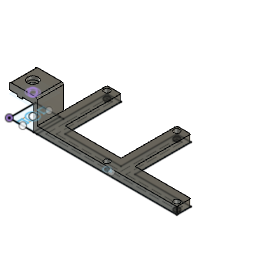
Micron_4010_Bed_FAN v2 (Autodesk Fusion 360 design; units mm, degrees)
Autodesk Fusion 360 part; units mm, degrees
sketch "Skizze1" plane through (0, 0, 0) normal (0, 0, 1) x (1, 0, 0)
  line L0 (0, 0) -> (0, 15)
  line L1 (0, 15) -> (14, 15)
  line L2 (14, 15) -> (14, 0)
  line L3 (14, 0) -> (0, 0)
  line L4 (14, 15) -> (16, 15)
  line L5 (14, 0) -> (16, 0)
  line L6 (16, 15) -> (16, 0)
  line L7 (16, 0) -> (96, 0)
  line L8 (96, 0) -> (96, 8)
  line L9 (16, 15) -> (16, 40)
  line L10 (16, 40) -> (24, 40)
  line L11 (24, 40) -> (24, 8)
  line L12 (24, 8) -> (56, 8)
  line L13 (56, 8) -> (56, 40)
  line L14 (56, 40) -> (64, 40)
  line L15 (64, 40) -> (64, 8)
  line L16 (64, 8) -> (96, 8)
  line L17 (18.5, 15) -> (18.5, 2.5) construction
  line L18 (18.5, 2.5) -> (93.5, 2.5) construction
  line L19 (93.5, 2.5) -> (93.5, 5.5) construction
  line L20 (61.5, 5.5) -> (93.5, 5.5) construction
  line L21 (61.5, 37.5) -> (61.5, 5.5) construction
  line L22 (58.5, 37.5) -> (61.5, 37.5) construction
  line L23 (58.5, 5.5) -> (58.5, 37.5) construction
  line L24 (21.5, 5.5) -> (58.5, 5.5) construction
  line L25 (21.5, 37.5) -> (21.5, 5.5) construction
  line L26 (18.5, 37.5) -> (21.5, 37.5) construction
  line L27 (18.5, 15) -> (18.5, 37.5) construction
  circle A0 centre (18.5, 37.5) radius 1.675
  circle A1 centre (58.5, 37.5) radius 1.675
  circle A2 centre (93.5, 2.5) radius 1.675
  line L28 (4.25, 0) -> (4.25, 15) construction
  line L29 (7.75, 0) -> (7.75, 15) construction
  line L30 (4.25, 0) -> (7.75, 0)
  line L31 (7.75, 0) -> (7.75, 3)
  line L32 (7.75, 3) -> (4.25, 3)
  line L33 (4.25, 3) -> (4.25, 0)
  line L34 (4.25, 15) -> (7.75, 15)
  line L35 (7.75, 15) -> (7.75, 12)
  line L36 (7.75, 12) -> (4.25, 12)
  line L37 (4.25, 12) -> (4.25, 15)
  circle A3 centre (6, 7.5) radius 1.5
  circle A4 centre (6, 7.5) radius 3
  line L38 (56, 2.5) -> (53.5, 2.5)
  circle A5 centre (53.5, 2.5) radius 1.675
  dimension "d1" = 15
  dimension "d2" = 14
  dimension "d3" = 2
  dimension "d4" = 2
  dimension "d5" = 80
  dimension "d6" = 8
  dimension "d7" = 90
  dimension "d8" = 25
  dimension "d9" = 90
  dimension "d10" = 8
  dimension "d11" = 32
  dimension "d12" = 32
  dimension "d13" = 32
  dimension "d14" = 8
  dimension "d15" = 90
  dimension "d16" = 32
  dimension "d17" = -2.5
  dimension "d18" = 3.35
  dimension "d20" = 3.35
  dimension "d21" = 3.35
  dimension "d26" = 3.5
  dimension "d27" = 3
  dimension "d28" = 3.5
  dimension "d29" = 3
  dimension "d30" = 3
  dimension "d31" = 6
  dimension "d64" = 2.5
  dimension "d65" = 3.35
  constraint coincident L0.start L3.end
  constraint vertical L0
  constraint perpendicular L0 L1
  constraint perpendicular L1 L2
  constraint perpendicular L0 L3
  constraint perpendicular L2 L4
  constraint perpendicular L2 L5
  constraint perpendicular L6 L7
  constraint perpendicular L4 L9
  constraint perpendicular L10 L11
  constraint perpendicular L11 L12
  constraint perpendicular L12 L13
  constraint perpendicular L14 L15
  constraint coincident L26.start L27.end
  constraint coincident L22.start L23.end
  constraint coincident L18.end L19.start
  constraint horizontal L30
  constraint vertical L31
  constraint horizontal L32
  constraint vertical L33
  constraint horizontal L34
  constraint vertical L35
  constraint horizontal L36
  constraint vertical L37
  constraint concentric A3 A4
  constraint parallel L18 L38
  constraint coincident L38.end A5.centre
  measures "d1" distance of L0.start L0.end
  measures "d2" distance of L0.end L1.end
  measures "d3" distance of L1.end L4.end
  measures "d4" distance of L2.end L5.end
  measures "d5" distance of L5.end L7.end
  measures "d6" distance of L7.end L8.end
  measures "d7" angle of L7 L8
  measures "d8" distance of L4.end L9.end
  measures "d9" angle of L9 L10
  measures "d10" distance of L9.end L10.end
  measures "d11" distance of L10.end L11.end
  measures "d12" distance of L11.end L12.end
  measures "d13" distance of L12.end L13.end
  measures "d14" distance of L13.end L14.end
  measures "d15" angle of L13 L14
  measures "d16" distance of L14.end L15.end
  measures "d18" diameter of A0
  measures "d20" diameter of A1
  measures "d21" diameter of A2
  measures "d26" distance of L28.start L29.start
  measures "d27" distance of L28.start L32.end
  measures "d28" distance of L28.end L29.end
  measures "d29" distance of L28.end L36.end
  measures "d30" diameter of A3
  measures "d31" diameter of A4
  measures "d64" distance of L38.start L38.end
  measures "d65" diameter of A5
extrude "Extrusion1" add sketch "Skizze1" along normal blind 4 contours L6 L7 L8 L9 L10 L11 L12 L13 L14 L15 L16 | A5 makes body 1
extrude "Extrusion2" add sketch "Skizze1" along normal blind 18 contours L2 L4 L5 L6 bodies 1
extrude "Extrusion3" add sketch "Skizze1" along normal blind 12 separate body contours L0 L1 L2 L3 L31 L32 L33 L35 L36 L37 | L3 L30 L31 L32 L33 | L1 L34 L35 L36 L37 | A3 | A4 makes body 2
sketch "Skizze2" plane through (0, 0, 12) normal (0, 0, 1) x (-1, 0, 0)
  line L0 (0, 0) -> (-14, 0)
  line L1 (-14, 0) -> (-14, -15)
  line L2 (-14, -15) -> (0, -15)
  line L3 (0, -15) -> (0, 0)
  circle A0 centre (-6, -7.5) radius 3
  circle A1 centre (-6, -7.5) radius 1.5
extrude "Extrusion4" cut sketch "Skizze1" along normal blind 8 contours L0 L1 L2 L3 L31 L32 L33 L35 L36 L37 bodies 2
extrude "Extrusion5" cut sketch "Skizze1" along normal blind 7 contours L3 L30 L31 L32 L33 | L1 L34 L35 L36 L37 bodies 2
extrude "Extrusion6" cut sketch "Skizze2" against normal blind 12 contours A1 bodies 2
extrude "Extrusion7" cut sketch "Skizze1" along normal blind 8 contours A4 bodies 2
extrude "Extrusion8" cut sketch "Skizze2" against normal blind 2 contours A0 bodies 2
move_face "Flächen versetzen1" offset -0.1 4 faces at (4.25, 2, 7.3333) (7.75, 1, 7.3333) (4.25, 13, 7.3333) (7.75, 14, 7.3333) on bodies 2
combine "Kombinieren1" operation add target body 1 tool bodies 2
fillet "Abrundung1" radius 0.5 9 edges at (56, 8, 2) (56, 40, 2) (64, 40, 2) (64, 8, 2) (96, 8, 2) (24, 40, 2) (16, 40, 2) (24, 8, 2) (96, 0, 2) on bodies 1
fillet "Abrundung2" radius 1 2 edges at (0, 7.5, 12) (16, 7.5, 18) on bodies 1
fillet "Abrundung3" radius 0.5 2 edges at (0, 7.5, 8) (14, 7.5, 8) on bodies 1
fillet "Abrundung4" radius 0.5 1 edges at (14, 7.5, 0) on bodies 1
fillet "Abrundung5" radius 0.5 1 edges at (16, 15, 2) on bodies 1
chamfer "Fase1" distance 1 angle 45 2 edges at (6, 12, 7) (6, 3, 7) on bodies 1
fillet "Abrundung6" radius 1 2 edges at (6, 2, 7) (6, 13, 7) on bodies 1
fillet "Abrundung7" radius 0.2 12 edges at (4.35, 2.6464, 7.6464) (4.35, 1.9685, 7.0761) (4.35, 0.7929, 7) (7.65, 0.7929, 7) (7.65, 1.9685, 7.0761) (7.65, 2.6464, 7.6464) (4.35, 14.2071, 7) (4.35, 13.0315, 7.0761) (4.35, 12.3536, 7.6464) (7.65, 12.3536, 7.6464) (7.65, 13.0315, 7.0761) (7.65, 14.2071, 7) on bodies 1
ref_plane "Arbeitsebene1" through (14, 7.5, 9) normal (-1, 0, 0) x (0, -1, 0)
split "Teilen1" by plane through (14, 7.5, 9) normal (-1, 0, 0) bodies 1 makes body 3 at (11.5, 7.5, 8)
move_body "Verschieben1" bodies 3 to x (1, 0, 0) y (0, 1, 0) z (0, 0, 1) at (0, 0, 6)
combine "Kombinieren2" operation add target body 1 tool bodies 3
extrude "Extrusion9" cut sketch "Skizze1" along normal blind 4 contours A5 bodies 1
move_face "Flächen versetzen2" offset -0.2 4 faces at (4.35, 0.5287, 13.4667) (4.35, 14.4713, 13.4667) (7.65, 14.4713, 13.4667) (7.65, 0.5287, 13.4667) on bodies 1
equation "d46 = 0.00 mm - 2 mm"
